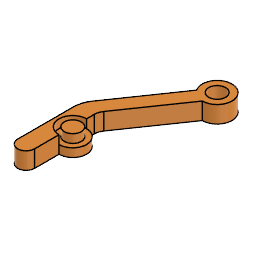
Lever (Autodesk Fusion 360 design; units mm, degrees)
part number: 2026-05-31-23-54-49-579
Autodesk Fusion 360 part; units mm, degrees
sketch "Sketch1" plane through (0, 0, 0) normal (0, 0, 1) x (1, 0, 0)
  circle A0 centre (0, 0) radius 2
  circle A1 centre (0, 0) radius 3.5
  circle A2 centre (-10, -24) radius 2
  circle A3 centre (-10, -24) radius 3.25
  line L0 (-10, -24) -> (-10, -20.75) construction
  line L1 (-10, -20.75) -> (-10, -18.9342)
  line L2 (0, 0) -> (0, -3.5) construction
  line L3 (-9.4696, -17.231) -> (0, -3.5)
  line L4 (-10, -24) -> (-10, -27.25) construction
  line L5 (-10, -27.25) -> (-10, -33)
  circle A4 centre (-12, -33) radius 2
  line L6 (-14, -33) -> (-14, -19.8683)
  line L7 (-12.9393, -16.462) -> (-2.9185, -1.9319)
  arc A5 (-12.9393, -16.462) -> (-14, -19.8683) centre (-8, -19.8683) ccw
  arc A6 (-9.4696, -17.231) -> (-10, -18.9342) centre (-7, -18.9342) ccw
  point P0 (-10, -18)
  point P1 (-14, -18)
  dimension "d1" = 4
  dimension "d2" = 7
  dimension "d3" = 4
  dimension "d4" = 24
  dimension "d5" = 10
  dimension "d6" = 6.5
  dimension "d7" = 2.75
  dimension "d8" = 4
  dimension "d9" = 5.75
  dimension "d11" = 15
  dimension "d12" = 4
  dimension "d13" = 6
  dimension "d14" = 3
  constraint coincident A0.centre A1.centre
  constraint concentric A0 A1
  constraint concentric A2 A3
  constraint coincident A2.centre A3.centre
  constraint coincident A3 L0.end
  constraint vertical L0
  constraint parallel L0 L1
  constraint coincident A1 L2.end
  constraint vertical L2
  constraint coincident A3 L4.end
  constraint parallel L0 L4
  constraint parallel L4 L5
  constraint coincident L5.end A4
  constraint tangent L5 A4
  constraint coincident A4 L6.start
  constraint parallel L1 L6
  constraint parallel L3 L7
  constraint coincident A1 L7.end
  constraint coincident P1 L6
  constraint coincident P1 L7
  constraint tangent L6 A5
  constraint tangent L7 A5
  constraint coincident P0 L1
  constraint coincident P0 L3
  constraint tangent L1 A6
  constraint tangent L3 A6
  measures "d1" diameter of A0
  measures "d2" diameter of A1
  measures "d3" diameter of A2
  measures "d4" vertical distance of A0.centre A2.centre
  measures "d5" horizontal distance of A0.centre A2.centre
  measures "d6" diameter of A3
  measures "d7" distance of L0.end P0
  measures "d8" diameter of A4
  measures "d9" distance of L4.end L5.end
  measures "d11" distance of L6.start P1
  measures "d12" distance of L5 L6
  measures "d13" radius of A5
  measures "d14" radius of A6
extrude "Extrude1" add sketch "Sketch1" along normal blind 4 contours A1 | A1 A3 L1 L3 L5 A4 L6 L7 A5 A6 | A4
extrude "Extrude2" add sketch "Sketch1" along normal blind 2 contours A3
extrude "Extrude3" add sketch "Sketch1" along normal blind 4 contours A2
